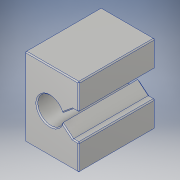
# Autodesk Inventor part: Führungswagen
Saved by Autodesk Inventor 2019 (Build 230136000, 136)
## iProperties
Created: 2021-05-01
Part Number: Führungswagen
Material: Aluminium 6061
Document SubType Name: Modeling
Designer: Michael Sumper
Density: 2.7 g/cm^3
Appearance: Aluminium - flach
Author: Michael Sumper
Autodesk Inventor part; units mm, degrees
ref_plane "YZ Plane" through (0, 0, 0) normal (1, 0, 0) x (0, 1, 0)
ref_plane "XZ Plane" through (0, 0, 0) normal (0, 1, 0) x (-1, 0, 0)
ref_plane "XY Plane" through (0, 0, 0) normal (0, 0, 1) x (1, 0, 0)
sketch "Skizze1" plane through (0, 0, 0) normal (0, 0, 1) x (1, 0, 0)
  line L0 (13.8, 20) -> (-13.8, 20)
  line L1 (-13.8, 20) -> (-13.8, -20)
  line L2 (-13.8, -20) -> (13.8, -20)
  line L3 (13.8, 20) -> (-13.8, -20) construction
  line L4 (-13.8, 20) -> (13.8, -20) construction
  line L5 (13.8, 20) -> (13.8, 6.65) construction
  line L6 (13.8, 6.65) -> (10.7, 6.65)
  line L7 (-13.8, 0) -> (-0.95, 0) construction
  arc A0 (5.3287, 2.1909) -> (5.3287, -2.1909) centre (-0.95, 0) ccw
  line L8 (10.7, 6.65) -> (5.3287, 2.1909)
  line L9 (13.8, 6.65) -> (13.8, -6.65) construction
  line L10 (13.8, -6.65) -> (10.7, -6.65)
  line L11 (10.7, -6.65) -> (5.3287, -2.1909)
  line L12 (13.8, -20) -> (13.8, -6.65)
  line L13 (13.8, 6.65) -> (13.8, 20)
  point P0 (0, 0)
  dimension "d0" = 27.6
  dimension "d1" = 40
  dimension "d2" = 13.35
  dimension "d3" = 3.1
  dimension "d4" = 12.85
  dimension "d5" = 13.3
  dimension "d6" = 6.981
  dimension "d7" = 13.3
  dimension "d8" = 3.1
  dimension "d9" = 6.981
  constraints: 28 end point, 4 perpendicular, 3 horizontal, 3 midpoint, 3 parallel, 2 point on circle, 1 centre point, 1 coincident
  measures "d0" distance of L2.end L1.end
  measures "d1" distance of L1.end L0.end
  measures "d2" distance of L0.start L5.end
  measures "d3" distance of L5.end L6.end
  measures "d4" distance of L7.start L7.end
  measures "d5" diameter of A0
  measures "d6" distance of L6.end L8.end
  measures "d7" distance of L5.end L9.end
  measures "d8" distance of L9.end L10.end
  measures "d9" distance of L10.end L11.end
extrude "Extrusion1" add sketch "Skizze1" along normal blind 39
sketch "Skizze2" plane through (-13.8, -20, 0) normal (-1, 0, 0) x (0, 0, 1)
  line L0 (0, 40) -> (39, 40) construction
  line L1 (0, 0) -> (39, 0) construction
  line L2 (0, 40) -> (39, 0) construction
  line L3 (39, 40) -> (0, 0) construction
  line L4 (6.5, 6) -> (32.5, 6) construction
  line L5 (32.5, 6) -> (32.5, 34) construction
  line L6 (32.5, 34) -> (6.5, 34) construction
  line L7 (6.5, 34) -> (6.5, 6) construction
  line L8 (6.5, 6) -> (32.5, 34) construction
  line L9 (32.5, 6) -> (6.5, 34) construction
  point P0 (0, 20)
  point P1 (19.5, 20)
  dimension "d12" = 26
  dimension "d13" = 28
  constraints: 16 end point, 3 midpoint, 2 parallel, 1 horizontal, 1 perpendicular
  measures "d12" distance of L6.end L5.end
  measures "d13" distance of L5.end L4.end
hole "Bohrung1" at (-13.8, 14, 6.5) at (-13.8, 14, 32.5) at (-13.8, -14, 32.5) at (-13.8, -14, 6.5) direction (1, 0, 0) diameter 3.242 depth 11.8 tip angle 118 thread size "M4x0.7" class "6H" standard "ANSI Metric M Profile"
chamfer "Fase1" distance 0.5 angle 45 26 edges at (13.8, 13.325, 39) (13.8, 13.325, 0) (13.8, -13.325, 0) (13.8, -13.325, 39) (13.8, -20, 19.5) (0, -20, 39) (-13.8, 0, 39) (0, 20, 39) (-13.8, 20, 19.5) (0, 20, 0) (13.8, 6.65, 19.5) (13.8, -6.65, 19.5) (-7.6, 0, 39) (8.0144, -4.4204, 39) (12.25, -6.65, 39) (8.0144, 4.4204, 39) (12.25, 6.65, 39) (-7.6, 0, 0) (8.0144, -4.4204, 0) (12.25, -6.65, 0) (12.25, 6.65, 0) (8.0144, 4.4204, 0) (0, -20, 0) (-13.8, -20, 19.5) (-13.8, 0, 0) (13.8, 20, 19.5)
